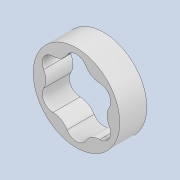
# Autodesk Inventor part: 1ギア接続部外
Saved by Autodesk Inventor 2020.4 (Build 244396000, 396)
## iProperties
Created: 2021-04-23
Part Number: 1ギア接続部外
Material: アルミニウム 2014-T4
Document SubType Name: Modeling
Designer: happy
Density: 2.8 g/cm^3
Appearance: サテン
Author: happy
Autodesk Inventor part; units mm, degrees
ref_plane "YZ Plane" through (0, 0, 0) normal (1, 0, 0) x (0, 1, 0)
ref_plane "XZ Plane" through (0, 0, 0) normal (0, 1, 0) x (-1, 0, 0)
ref_plane "XY Plane" through (0, 0, 0) normal (0, 0, 1) x (1, 0, 0)
sketch "スケッチ1" plane through (0, 0, 0) normal (0, 0, 1) x (1, 0, 0)
  circle A0 centre (45.6488, -28.0072) radius 8
  circle A1 centre (45.6488, -28.0072) radius 7 construction
  line L0 (45.6488, -21.0072) -> (51.7109, -24.5072) construction
  line L1 (51.7109, -24.5072) -> (51.7109, -31.5072) construction
  line L2 (51.7109, -31.5072) -> (45.6488, -35.0072) construction
  line L3 (45.6488, -35.0072) -> (39.5866, -31.5072) construction
  line L4 (39.5866, -31.5072) -> (39.5866, -24.5072) construction
  line L5 (39.5866, -24.5072) -> (45.6488, -21.0072) construction
  arc A2 (47.3808, -22.0072) -> (43.9167, -22.0072) centre (45.6488, -23.0072) ccw
  arc A3 (41.3186, -23.5072) -> (39.5866, -26.5072) centre (41.3186, -25.5072) ccw
  arc A4 (39.5866, -29.5072) -> (41.3186, -32.5072) centre (41.3186, -30.5072) ccw
  arc A5 (43.9167, -34.0072) -> (47.3808, -34.0072) centre (45.6488, -33.0072) ccw
  arc A6 (49.9789, -32.5072) -> (51.7109, -29.5072) centre (49.9789, -30.5072) ccw
  arc A7 (51.7109, -26.5072) -> (49.9789, -23.5072) centre (49.9789, -25.5072) ccw
  arc A8 (47.3808, -22.0072) -> (49.9789, -23.5072) centre (49.9789, -20.5072) ccw
  arc A9 (41.3186, -23.5072) -> (43.9167, -22.0072) centre (41.3186, -20.5072) ccw
  arc A10 (39.5866, -29.5072) -> (39.5866, -26.5072) centre (36.9885, -28.0072) ccw
  arc A11 (43.9167, -34.0072) -> (41.3186, -32.5072) centre (41.3186, -35.5072) ccw
  arc A12 (49.9789, -32.5072) -> (47.3808, -34.0072) centre (49.9789, -35.5072) ccw
  arc A13 (51.7109, -26.5072) -> (51.7109, -29.5072) centre (54.309, -28.0072) ccw
  circle A14 centre (45.6488, -28.0072) radius 5.6603 construction
  point P0 (0, 0)
  point P1 (51.7109, -31.5072)
  point P2 (51.7109, -24.5072)
  point P3 (39.5866, -26.5072)
  point P4 (41.3186, -23.5072)
  point P5 (43.9167, -22.0072)
  point P6 (51.7109, -26.5072)
  dimension "d5" = 14
  dimension "d4" = 16
  dimension "d6" = 360
  dimension "d7" = 360
  dimension "d8" = 11.3205
  dimension "d9" = 3
  dimension "d10" = 2
  constraints: 30 point on circle, 14 centre point, 12 end point, 3 coincident, 2 point on line, 2 tangent, 1 vertical, 1 vertical alignment, 73 other
  measures "d4" diameter of A0
  measures "d8" diameter of A14
  measures "d9" radius of A8
  measures "d10" radius of A2
extrude "押し出し1" add sketch "スケッチ1" along normal blind 5
